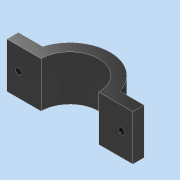
# Autodesk Inventor part: Part3
Saved by Autodesk Inventor 2022 (Build 260153000, 153)
## iProperties
Created: 2022-09-15
Part Number: Part3
Material: Generic
Document SubType Name: Modeling
Designer: aleal
Density: 1 g/cm^3
Appearance: Glossy - Black
Author: aleal
Autodesk Inventor part; units mm, degrees
ref_plane "YZ Plane" through (0, 0, 0) normal (1, 0, 0) x (0, 1, 0)
ref_plane "XZ Plane" through (0, 0, 0) normal (0, 1, 0) x (-1, 0, 0)
ref_plane "XY Plane" through (0, 0, 0) normal (0, 0, 1) x (1, 0, 0)
sketch "Sketch1" plane through (0, 0, 0) normal (0, 1, 0) x (-1, 0, 0)
  arc A0 (-25.4, 0) -> (25.4, 0) centre (0, 0) ccw
  arc A1 (-35.4, 0) -> (35.4, 0) centre (0, 0) ccw
  line L0 (-35.4, 0) -> (-25.4, 0)
  line L1 (25.4, 0) -> (35.4, 0)
  line L2 (35.4, 0) -> (55.4, 0)
  line L3 (55.4, 0) -> (55.4, -10)
  line L4 (55.4, -10) -> (33.9582, -10)
  line L5 (-35.4, 0) -> (-55.4, 0)
  line L6 (-55.4, 0) -> (-55.4, -10)
  line L7 (-55.4, -10) -> (-33.9582, -10)
  dimension "d0" = 50.8
  dimension "d1" = 10
  dimension "d2" = 20
  dimension "d3" = 10
  dimension "d4" = 20
  dimension "d5" = 10
  constraints: 16 end point, 6 point on circle, 4 horizontal, 4 perpendicular, 2 centre point, 1 coincident
  measures "d0" diameter of A0
  measures "d1" radial gap between concentric circles of A0 A1
  measures "d2" distance of L1.end L2.end
  measures "d3" distance of L2.end L3.end
  measures "d4" distance of L0.start L5.end
  measures "d5" distance of L5.end L6.end
extrude "Extrusion1" add sketch "Sketch1" along normal blind 40
sketch "Sketch2" plane through (-55.4, 0, 0) normal (0, 0, 1) x (1, 0, 0)
  circle A0 centre (10, 20) radius 2.75
  circle A1 centre (100.8, 20) radius 2.75
  line L0 (80.8, 40) -> (110.8, 40) projected
  line L1 (110.8, 0) -> (110.8, 40) projected
  line L2 (0, 0) -> (0, 40) projected
  line L3 (0, 40) -> (30, 40) projected
  point P0 (55.4, 0)
  dimension "d8" = 5.5
  dimension "d9" = 5.5
  dimension "d10" = 20
  dimension "d11" = 10
  dimension "d12" = 10
  dimension "d13" = 20
  constraints: 2 centre point
  measures "d8" diameter of A0
  measures "d9" diameter of A1
  measures "d10" distance from line of L0 A1.centre
  measures "d11" distance from line of L1 A1.centre
  measures "d12" distance from line of L2 A0.centre
  measures "d13" distance from line of L3 A0.centre
extrude "Extrusion2" cut sketch "Sketch2" against normal blind 40
body "Solid1"
